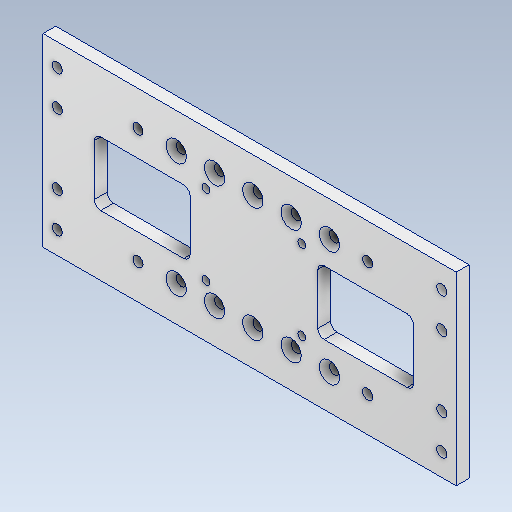
# Autodesk Inventor part: 조인트3받침_6T
Saved by Autodesk Inventor 2020.5 (Build 245400000, 400)
## iProperties
Created: 2022-01-24
Part Number: 조인트3받침_6T
Material: 알루미늄 6061
Document SubType Name: Modeling
Designer: BAEK
Density: 2.7 g/cm^3
Appearance: 알루미늄 - 평지
Mass: 65.6468 g
Surface Area: 154.646 cm^2
Volume: 24.3136 cm^3
Author: BAEK
Autodesk Inventor part; units mm, degrees
ref_plane "YZ Plane" through (0, 0, 0) normal (1, 0, 0) x (0, 1, 0)
ref_plane "XZ Plane" through (0, 0, 0) normal (0, 1, 0) x (-1, 0, 0)
ref_plane "XY Plane" through (0, 0, 0) normal (0, 0, 1) x (1, 0, 0)
sketch "스케치1" plane through (0, 0, 0) normal (0, 0, 1) x (1, 0, 0)
  line L0 (0, 0) -> (0, 58)
  line L1 (0, 58) -> (129.5, 58)
  line L2 (129.5, 58) -> (129.5, 0)
  line L3 (129.5, 0) -> (0, 0)
  dimension "d0" = 58
  dimension "d1" = 129.5
  constraints: 8 end point, 3 perpendicular, 1 vertical
  measures "d0" distance of L0.start L0.end
  measures "d1" distance of L0.end L1.end
extrude "돌출1" add sketch "스케치1" along normal blind 4
sketch "스케치2" plane through (0, 0, 4) normal (0, 0, 1) x (1, 0, 0)
  line L0 (62.75, 50) -> (62.75, 8)
  line L1 (32.75, 50) -> (57.25, 50)
  line L2 (62.75, 50) -> (69.25, 50)
  line L3 (81.25, 8) -> (81.25, 50)
  line L4 (74.75, 50) -> (81.25, 50)
  line L5 (74.75, 50) -> (74.75, 8)
  line L6 (74.75, 8) -> (81.25, 8)
  circle A0 centre (77.75, 47) radius 1.6
  circle A1 centre (77.75, 11) radius 1.6
  line L7 (93.25, 8) -> (93.25, 50)
  line L8 (86.75, 50) -> (93.25, 50)
  line L9 (86.75, 50) -> (86.75, 8)
  line L10 (86.75, 8) -> (93.25, 8)
  circle A2 centre (89.75, 47) radius 1.6
  circle A3 centre (89.75, 11) radius 1.6
  line L11 (57.25, 8) -> (57.25, 50)
  line L12 (32.75, 50) -> (57.25, 50)
  line L13 (32.75, 50) -> (32.75, 54)
  line L14 (26.75, 54) -> (32.75, 54)
  line L15 (26.75, 4) -> (26.75, 54)
  line L16 (26.75, 4) -> (32.75, 4)
  line L17 (32.75, 4) -> (32.75, 8)
  line L18 (32.75, 8) -> (57.25, 8)
  circle A4 centre (29.75, 47) radius 1.6
  circle A5 centre (29.75, 11) radius 1.6
  circle A6 centre (41.75, 47) radius 1.6
  circle A7 centre (41.75, 11) radius 1.6
  circle A8 centre (53.75, 47) radius 1.6
  circle A9 centre (53.75, 11) radius 1.6
  line L19 (62.75, 8) -> (69.25, 8)
  circle A10 centre (65.75, 47) radius 1.6
  circle A11 centre (65.75, 11) radius 1.6
  circle A12 centre (101.75, 11) radius 1.6
  circle A13 centre (113.75, 11) radius 1.6
  circle A14 centre (113.75, 47) radius 1.6
  circle A15 centre (101.75, 47) radius 1.6
  circle A16 centre (5.75, 11) radius 1.6
  circle A17 centre (5.75, 47) radius 1.6
  line L20 (113.75, 11) -> (113.75, 47)
  line L21 (5.75, 11) -> (5.75, 47)
  line L22 (129.5, 0) -> (129.5, 58) projected
  line L23 (0, 0) -> (129.5, 0) projected
  line L24 (0, 58) -> (0, 0) projected
  line L25 (113.75, 47) -> (132.75, 47)
  line L26 (113.75, 11) -> (132.75, 11)
  line L27 (132.75, 11) -> (132.75, 47)
  line L28 (5.75, 47) -> (-3.25, 47)
  line L29 (-3.25, 47) -> (-3.25, 11)
  line L30 (-3.25, 11) -> (5.75, 11)
  line L31 (-3.25, 29) -> (132.75, 29)
  line L32 (0, 58) -> (-3.25, 58)
  line L33 (-3.25, 58) -> (-3.25, 0)
  line L34 (-3.25, 0) -> (0, 0)
  dimension "d27" = 19
  dimension "d28" = 9
  dimension "d30" = 3.25
  dimension "d31" = 21
  dimension "d32" = 5.5
  dimension "d34" = 3.25
  constraints: 64 end point, 18 centre point, 5 perpendicular, 3 horizontal, 2 midpoint, 1 vertical, 2 other
  measures "d27" distance of L20.end L25.end
  measures "d28" distance of L21.end L28.end
  measures "d30" distance between parallel lines of L27 L22
  measures "d31" distance between parallel lines of L15 L21
  measures "d32" distance between parallel lines of L0 L11
  measures "d34" distance of the line from the sketch origin of L29
extrude "돌출2" cut sketch "스케치2" against normal blind 6 contours L21 L30 A16 | A16 L30 L21 | L21 L28 A17 | A17 L28 L21 | L20 L26 A13 | A13 L26 L20 | L20 L25 A14 | A14 L25 L20 | A0 | A1 | A2 | A3 | A4 | A5 | A6 | A7 | A8 | A9 | A10 | A11 | A12 | A15
sketch "스케치3" plane through (0, 0, 4) normal (0, 0, 1) x (1, 0, 0)
  circle A0 centre (29.75, 47) radius 1.6 projected
  circle A1 centre (41.75, 11) radius 1.6 projected
  circle A2 centre (89.75, 11) radius 1.6 projected
  circle A3 centre (101.75, 47) radius 1.6 projected
  circle A4 centre (113.75, 11) radius 1.6 projected
  circle A5 centre (89.75, 47) radius 1.6 projected
  circle A6 centre (77.75, 11) radius 1.6 projected
  circle A7 centre (29.75, 11) radius 1.6 projected
  circle A8 centre (5.75, 47) radius 1.6 projected
  circle A9 centre (41.75, 47) radius 1.6 projected
  circle A10 centre (53.75, 11) radius 1.6 projected
  circle A11 centre (65.75, 47) radius 1.6 projected
  circle A12 centre (113.75, 47) radius 1.6 projected
  circle A13 centre (101.75, 11) radius 1.6 projected
  circle A14 centre (77.75, 47) radius 1.6 projected
  circle A15 centre (65.75, 11) radius 1.6 projected
  circle A16 centre (53.75, 47) radius 1.6 projected
  circle A17 centre (5.75, 11) radius 1.6 projected
  line L0 (129.5, 58) -> (0, 58) projected
  line L1 (0, 58) -> (0, 0) projected
  line L2 (0, 0) -> (129.5, 0) projected
  line L3 (129.5, 0) -> (129.5, 58) projected
extrude "돌출3" add sketch "스케치3" against normal blind 4 contours A4 | A8 | A12 | A17
sketch "스케치4" plane through (0, 0, 4) normal (0, 0, 1) x (1, 0, 0)
  line L0 (129.5, 58) -> (0, 58) projected
  line L1 (4.5, 58) -> (4.5, 0) construction
  line L2 (0, 0) -> (129.5, 0) projected
  line L3 (0, 58) -> (0, 0) projected
  line L4 (64.75, 58) -> (64.75, 0) construction
  circle A0 centre (4.5, 51) radius 1.6
  circle A1 centre (4.5, 40) radius 1.6
  circle A2 centre (4.5, 18) radius 1.6
  circle A3 centre (4.5, 7) radius 1.6
  circle A4 centre (125, 51) radius 1.6
  circle A5 centre (125, 40) radius 1.6
  circle A6 centre (125, 18) radius 1.6
  circle A7 centre (125, 7) radius 1.6
  dimension "d10" = 4.5
  dimension "d11" = 3.2
  dimension "d12" = 3.2
  dimension "d13" = 3.2
  dimension "d14" = 3.2
  dimension "d15" = 11
  dimension "d16" = 22
  dimension "d17" = 11
  dimension "d18" = 7
  constraints: 8 centre point, 6 point on line, 4 end point, 4 symmetric about line, 2 midpoint, 1 vertical, 4 other
  measures "d10" distance between parallel lines of L3 L1
  measures "d11" diameter of A0
  measures "d12" diameter of A1
  measures "d13" diameter of A2
  measures "d14" diameter of A3
  measures "d15" distance of A0.centre A1.centre
  measures "d16" distance of A2.centre A1.centre
  measures "d17" distance of A2.centre A3.centre
  measures "d18" distance from line of L2 A3.centre
extrude "돌출4" cut sketch "스케치4" against normal blind 4
sketch "스케치5" plane through (0, 0, 4) normal (0, 0, 1) x (1, 0, 0)
  line L0 (116.0982, 37) -> (116.0982, 21)
  line L1 (16.0982, 21) -> (16.0982, 37)
  line L2 (0, 0) -> (129.5, 0) projected
  arc A0 (18.0982, 39) -> (16.0982, 37) centre (18.0982, 37) ccw
  arc A1 (16.0982, 21) -> (18.0982, 19) centre (18.0982, 21) ccw
  arc A2 (116.0982, 37) -> (114.0982, 39) centre (114.0982, 37) ccw
  arc A3 (114.0982, 19) -> (116.0982, 21) centre (114.0982, 21) ccw
  line L3 (66.0982, 39) -> (66.0982, 19)
  line L4 (46.0982, 37) -> (46.0982, 21)
  line L5 (86.0982, 37) -> (86.0982, 21)
  line L6 (18.0982, 39) -> (44.0982, 39)
  line L7 (88.0982, 39) -> (114.0982, 39)
  line L8 (114.0982, 19) -> (88.0982, 19)
  line L9 (44.0982, 19) -> (18.0982, 19)
  arc A4 (46.0982, 37) -> (44.0982, 39) centre (44.0982, 37) ccw
  arc A5 (44.0982, 19) -> (46.0982, 21) centre (44.0982, 21) ccw
  arc A6 (86.0982, 21) -> (88.0982, 19) centre (88.0982, 21) ccw
  arc A7 (88.0982, 39) -> (86.0982, 37) centre (88.0982, 37) ccw
  point P0 (16.0982, 39)
  point P1 (116.0982, 19)
  point P2 (116.0982, 39)
  dimension "d35" = 100
  dimension "d36" = 20
  dimension "d38" = 2
  dimension "d41" = 20
  dimension "d42" = 20
  dimension "d43" = 2
  constraints: 20 tangent, 18 end point, 16 point on circle, 8 centre point, 7 parallel, 6 equal radius, 3 point on line, 2 horizontal, 2 perpendicular
  measures "d35" distance of point (16.098, 39) point (116.098, 39)
  measures "d36" distance of point (116.098, 39) point (116.098, 19)
  measures "d38" radius of A0
  measures "d41" distance between parallel lines of L3 L4
  measures "d42" distance between parallel lines of L3 L5
  measures "d43" radius of A4
extrude "돌출5" cut sketch "스케치5" against normal blind 4
sketch "스케치6" plane through (0, 0, 4) normal (0, 0, 1) x (1, 0, 0)
  line L0 (81.0982, 41.5) -> (81.0982, 16.5) construction
  line L1 (81.0982, 16.5) -> (51.0982, 16.5) construction
  line L2 (51.0982, 16.5) -> (51.0982, 41.5) construction
  line L3 (51.0982, 41.5) -> (81.0982, 41.5) construction
  circle A0 centre (81.0982, 41.5) radius 1.25
  circle A1 centre (81.0982, 16.5) radius 1.25
  circle A2 centre (51.0982, 41.5) radius 1.25
  circle A3 centre (51.0982, 16.5) radius 1.25
  line L4 (46.0982, 37) -> (46.0982, 21) projected
  line L5 (129.5, 58) -> (0, 58) projected
  point P0 (0, 0)
  point P1 (66.0982, 29)
  dimension "d44" = 25
  dimension "d45" = 30
  dimension "d46" = 15
  dimension "d47" = 12.5
  dimension "d48" = 2.5
  dimension "d49" = 2.5
  dimension "d50" = 2.5
  dimension "d51" = 2.5
  dimension "d52" = 5
  dimension "d53" = 16.5
  constraints: 8 end point, 4 centre point, 4 coincident, 2 parallel, 1 perpendicular
  measures "d44" distance of L1.end L2.end
  measures "d45" distance of L0.end L1.end
  measures "d46" distance from line of L0 point (66.098, 29)
  measures "d47" distance from line of point (66.098, 29) L1
  measures "d48" diameter of A0
  measures "d49" diameter of A1
  measures "d50" diameter of A2
  measures "d51" diameter of A3
  measures "d52" distance between parallel lines of L4 L2
  measures "d53" distance between parallel lines of L5 L3
extrude "돌출6" cut sketch "스케치6" against normal blind 10
chamfer "모따기1" distance 1.6 angle 45 10 edges at (52.15, 47, 4) (40.15, 47, 4) (64.15, 47, 4) (76.15, 47, 4) (88.15, 47, 4) (88.15, 11, 4) (76.15, 11, 4) (64.15, 11, 4) (52.15, 11, 4) (40.15, 11, 4)
